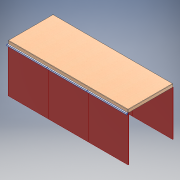
# Autodesk Inventor part: 1420-1+4-04 Table
Saved by Autodesk Inventor 2017 (Build 210142000, 142)
## iProperties
Company: FABLAB Frenchmakers
Part Number: 1420-1+4-04 Table
Project: 1420 VAUBAN 3D XL
Material: Générique
Catalog Web Link: http://www.frenchmakers.com/
Document SubType Name: Modeling
Designer: Adrien MARY
Mass: 105319 g
Surface Area: 95930.4 cm^2
Volume: 105319 cm^3
Density: 1 g/cm^3
Appearance: Chêne blanc - Massif lustre moyen naturel
Author: Adrien MARY
Autodesk Inventor part; units mm, degrees
ref_plane "YZ Plane" through (0, 0, 0) normal (1, 0, 0) x (0, 1, 0)
ref_plane "XZ Plane" through (0, 0, 0) normal (0, 1, 0) x (-1, 0, 0)
ref_plane "XY Plane" through (0, 0, 0) normal (0, 0, 1) x (1, 0, 0)
sketch "Esquisse1" plane through (0, 0, 0) normal (0, 0, 1) x (1, 0, 0)
  line L0 (-1000, -375) -> (1000, -375)
  line L1 (1000, -375) -> (1000, 375)
  line L2 (1000, 375) -> (-1000, 375)
  line L3 (-1000, 375) -> (-1000, -375)
  line L4 (-1000, -375) -> (1000, 375) construction
  line L5 (1000, -375) -> (-1000, 375) construction
  point P0 (0, 0)
  dimension "d0" = 2000
  dimension "d1" = 750
  constraints: 12 end point, 2 midpoint, 2 parallel, 1 horizontal, 1 perpendicular
  measures "d0" distance of L2.end L1.end
  measures "d1" distance of L1.end L0.end
extrude "Extrusion1" add sketch "Esquisse1" along normal blind 50
sketch "Esquisse3" plane through (-1000, -375, 0) normal (0, -1, 0) x (1, 0, 0)
  line L0 (0, -750) -> (666.6667, -750)
  line L1 (666.6667, -750) -> (666.6667, 0)
  line L2 (666.6667, 0) -> (0, 0)
  line L3 (0, 0) -> (0, -750)
  line L4 (0, 0) -> (2000, 0) construction
  line L5 (2000, 0) -> (2000, 50) construction
  line L6 (0, 50) -> (2000, 50) construction
  line L7 (0, 0) -> (0, 50) construction
  point P0 (1000, 0)
  dimension "d8" = 2000
  dimension "d9" = 666.6667
  dimension "d10" = 750
  constraints: 8 end point, 2 parallel, 1 horizontal, 1 perpendicular
  measures "d8" distance between parallel lines of L5 L7
  measures "d9" distance of L0.start L0.end
  measures "d10" distance of L2.end L0.start
extrude "Extrusion3" add sketch "Esquisse3" against normal blind 10 separate body
sketch "Esquisse4" plane through (-1000, -375, -750) normal (-1, 0, 0) x (0, 0, 1)
  line L0 (730, -20) -> (730, -15)
  line L1 (730, -15) -> (745, -15)
  line L2 (745, -15) -> (745, 0)
  line L3 (745, 0) -> (750, 0)
  line L4 (750, 0) -> (750, -19)
  line L5 (749, -20) -> (730, -20)
  line L6 (750, 0) -> (0, 0) projected
  line L7 (750, 750) -> (750, 0) projected
  arc A0 (749, -20) -> (750, -19) centre (749, -19) ccw
  point P0 (750, 375)
  point P1 (750, -20)
  dimension "d16" = 5
  dimension "d17" = 5
  dimension "d18" = 15
  dimension "d19" = 15
  dimension "d26" = 1
  constraints: 13 end point, 3 perpendicular, 2 collinear, 2 point on circle, 2 point on line, 2 tangent, 2 vertical, 1 centre point, 1 parallel
  measures "d16" distance between parallel lines of L4 L2
  measures "d17" distance of L0.start L0.end
  measures "d18" distance of L1.end L2.end
  measures "d19" distance of L0.end L1.end
  measures "d26" radius of A0
extrude "Extrusion4" add sketch "Esquisse4" against normal up to surface (666.6667 mm away) separate body
pattern_linear "Réseau rectangulaire1" count 3 spacing 668 along (1, 0, 0) of "Extrusion3" bodies 2
pattern_linear "Réseau rectangulaire2" count 3 spacing 668 along (1, 0, 0) of "Extrusion4" bodies 3
mirror "Symétrie3" about plane through (0, 0, 0) normal (0, 1, 0) of "Extrusion3", "Réseau rectangulaire1" bodies 2
fillet "Congé1" radius 5 7 edges at (0, -375, 50) (-1000, 0, 50) (-1000, -375, 25) (-1000, 375, 25) (0, 375, 50) (1000, -375, 25) (1000, 0, 50)
equation "\"d9\" = 0.333333 * d8"
